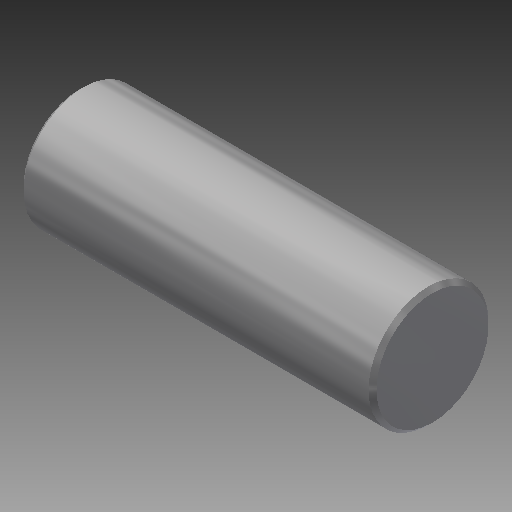
# Autodesk Inventor part: Eje silla - Interno
Saved by Autodesk Inventor 2019 (Build 230136000, 136)
## iProperties
Created: 2019-11-15
Part Number: Eje silla - Interno
Material: Steel
Document SubType Name: Modeling
Designer: Domenico
Density: 1 g/cm^3
Appearance: Steel
CustomPartVersion: 1
Author: Domenico
Autodesk Inventor part; units mm, degrees
ref_plane "Start Plane" through (0, 0, 0) normal (1, 0, 0) x (0, 1, 0)
ref_plane "XZ Plane" through (0, 0, 0) normal (0, 1, 0) x (-1, 0, 0)
ref_plane "XY Plane" through (0, 0, 0) normal (0, 0, 1) x (1, 0, 0)
sketch "Main Sketch" plane through (0, 0, 0) normal (0, 0, 1) x (1, 0, 0)
  line L0 (0, 0) -> (45, 0)
  line L1 (0, 0) -> (0, 7.65)
  line L2 (45, 7.65) -> (45, 0)
  line L3 (0, 7.65) -> (45, 7.65)
  dimension "d3" = 15.3
  constraints: 8 end point, 2 vertical, 1 horizontal
  measures "d3" diameter of L3 L0
revolve "Revolution1" add sketch "Main Sketch" angle 360 about axis through (0, 0, 0) along (1, 0, 0)
chamfer "Chamfer3" distance 0.5 angle 45 1 edges at (45, -7.65, 0) measured on face at (30, 7.5509, -1.2271)
chamfer "Chamfer2" distance 0.5 angle 45 1 edges at (0, -7.65, 0) measured on face at (14.8333, 7.6252, -0.6156)
body "Solid1"
